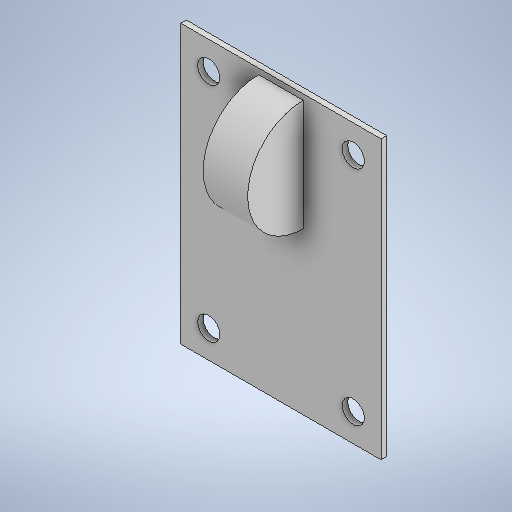
# Autodesk Inventor part: Placa-Circuito
Saved by Autodesk Inventor 2025 (Build 290162010, 162A)
## iProperties
Created: 2025-10-21
Part Number: Placa-Circuito
Material: Genérico
Document SubType Name: Modeling
Designer: 202321250026
Density: 1 g/cm^3
Appearance: Padrão
Author: 202321250026
Autodesk Inventor part; units mm, degrees
ref_plane "YZ Plane" through (0, 0, 0) normal (1, 0, 0) x (0, 1, 0)
ref_plane "XZ Plane" through (0, 0, 0) normal (0, 1, 0) x (-1, 0, 0)
ref_plane "XY Plane" through (0, 0, 0) normal (0, 0, 1) x (1, 0, 0)
sketch "Esboço1" plane through (0, 0, 0) normal (0, 0, 1) x (1, 0, 0)
  circle A0 centre (-13, -20) radius 2 projected
  circle A1 centre (-13, 20) radius 2 projected
  circle A2 centre (13, -20) radius 2 projected
  circle A3 centre (13, 20) radius 2 projected
  arc A4 (-15, 28) -> (-21, 22) centre (-15, 22) ccw projected
  line L0 (-21, 22) -> (-21, -38) projected
  arc A5 (-21, -38) -> (-15, -44) centre (-15, -38) ccw projected
  line L1 (-15, -44) -> (15, -44) projected
  arc A6 (15, -44) -> (21, -38) centre (15, -38) ccw projected
  line L2 (21, -38) -> (21, 22) projected
  arc A7 (21, 22) -> (15, 28) centre (15, 22) ccw projected
  line L3 (15, 28) -> (-15, 28) projected
  line L4 (-18, 25) -> (18, 25)
  line L5 (18, 25) -> (18, -25)
  line L6 (18, -25) -> (-18, -25)
  line L7 (-18, -25) -> (-18, 25)
  point P0 (0, 0)
  constraints: 8 end point, 2 parallel, 1 horizontal, 1 perpendicular
extrude "Extrusão1" add sketch "Esboço1" along normal blind 1 contours L4 L5 L6 L7
sketch "Esboço2" plane through (0, 0, 1) normal (0, 0, 1) x (1, 0, 0)
  line L0 (-4, 24) -> (4, 24)
  line L1 (4, 24) -> (4, 14)
  line L2 (4, 14) -> (-4, 14)
  line L3 (-4, 14) -> (-4, 24)
  circle A0 centre (-13, 20) radius 2 projected
  circle A1 centre (13, 20) radius 2 projected
  line L4 (18, 25) -> (-18, 25) projected
  point P0 (0, 0)
  dimension "d7" = 8
  dimension "d8" = 10
  dimension "d10" = 7
  dimension "d12" = 1
  constraints: 8 end point, 2 parallel, 1 horizontal, 1 perpendicular
  measures "d7" distance of L0.start L0.end
  measures "d8" distance of L2.end L0.start
  measures "d10" distance edge to line of A0 L3
  measures "d12" distance between parallel lines of L4 L0
revolve "Revolução1" add sketch "Esboço2" angle 180 about axis through (4, 14, 1) along (1, 0, 0) contours L0 L1 L2 L3
